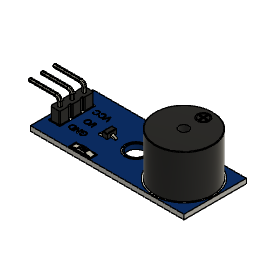
Buzzer (Autodesk Fusion 360 design; units mm, degrees)
Autodesk Fusion 360 part; units mm, degrees
note: some values were not read from the file. Set by a fixed rule: which face or edge a step refers to.
sketch "Sketch1" plane through (0, 0, 0) normal (0, 0, 1) x (1, 0, 0)
  line L0 (16, 6.5) -> (-16, 6.5)
  line L1 (-16, 6.5) -> (-16, -6.5)
  line L2 (-16, -6.5) -> (16, -6.5)
  line L3 (16, -6.5) -> (16, 6.5)
  line L4 (16, 6.5) -> (-16, -6.5) construction
  line L5 (-16, 6.5) -> (16, -6.5) construction
  dimension "d1" = 32
  dimension "d2" = 13
  constraint horizontal L0
  constraint perpendicular L0 L1
  constraint parallel L0 L2
  constraint parallel L1 L3
  constraint coincident L4 origin
  constraint coincident L5 origin
  measures "d1" distance of L1.end L2.end
  measures "d2" distance of L0.end L1.end
extrude "Extrude1" add sketch "Sketch1" along normal blind 1 makes body 1
sketch "Sketch2" plane through (0, 0, 1) normal (0, 0, 1) x (-1, 0, 0)
  line L0 (-16, 6.5) -> (-16, -6.5)
  line L1 (-16, -6.5) -> (16, -6.5)
  line L2 (16, -6.5) -> (16, 6.5)
  line L3 (16, 6.5) -> (-16, 6.5)
  circle A0 centre (-9.5, 0) radius 6
  line L4 (-9.5, 0) -> (-9.5, -6)
  line L5 (-9.5, 0) -> (-15.5, 0)
  circle A1 centre (0.5, 0) radius 1.75
  line L6 (5.5, 1) -> (6.5, 1)
  line L7 (6.5, 1) -> (6.5, -1)
  line L8 (6.5, -1) -> (5.5, -1)
  line L9 (5.5, -1) -> (5.5, 1)
  line L10 (5.5, 1) -> (6.5, -1) construction
  line L11 (6.5, 1) -> (5.5, -1) construction
  line L12 (6.5, 1) -> (7.5, 1)
  line L13 (7.5, 1) -> (7.5, 0.5)
  line L14 (7.5, 0.5) -> (6.5, 0.5)
  line L15 (6.5, 0.5) -> (6.5, 1)
  line L16 (6.5, -1) -> (7.5, -1)
  line L17 (7.5, -1) -> (7.5, -0.5)
  line L18 (7.5, -0.5) -> (6.5, -0.5)
  line L19 (6.5, -0.5) -> (6.5, -1)
  line L20 (5.5, 0.25) -> (4.5, 0.25)
  line L21 (4.5, 0.25) -> (4.5, -0.25)
  line L22 (4.5, -0.25) -> (5.5, -0.25)
  line L23 (5.5, -0.25) -> (5.5, 0.25)
  line L24 (4, 6) -> (8, 6)
  line L25 (8, 6) -> (8, 5)
  line L26 (8, 5) -> (4, 5)
  line L27 (4, 5) -> (4, 6)
  line L28 (6, 0) -> (6, 5.5)
  line L29 (4, 6) -> (5.25, 6)
  line L30 (5.25, 6) -> (5.25, 5)
  line L31 (8, 6) -> (6.75, 6)
  line L32 (6.75, 6) -> (6.75, 5)
  line L33 (14.325, 2.705) -> (13.675, 2.705)
  line L34 (13.675, 2.705) -> (13.675, 2.055)
  line L35 (13.675, 2.055) -> (14.325, 2.055)
  line L36 (14.325, 2.055) -> (14.325, 2.705)
  line L37 (14.325, 2.705) -> (13.675, 2.055) construction
  line L38 (13.675, 2.705) -> (14.325, 2.055) construction
  line L39 (13.675, -0.485) -> (14.325, -0.485)
  line L40 (14.325, -0.485) -> (14.325, 0.165)
  line L41 (14.325, 0.165) -> (13.675, 0.165)
  line L42 (13.675, 0.165) -> (13.675, -0.485)
  line L43 (13.675, -0.485) -> (14.325, 0.165) construction
  line L44 (14.325, -0.485) -> (13.675, 0.165) construction
  line L45 (13.675, -3.025) -> (14.325, -3.025)
  line L46 (14.325, -3.025) -> (14.325, -2.375)
  line L47 (14.325, -2.375) -> (13.675, -2.375)
  line L48 (13.675, -2.375) -> (13.675, -3.025)
  line L49 (13.675, -3.025) -> (14.325, -2.375) construction
  line L50 (14.325, -3.025) -> (13.675, -2.375) construction
  line L51 (15, 1.38) -> (13, 1.38)
  line L52 (13, 1.38) -> (13, 3.38)
  line L53 (13, 3.38) -> (15, 3.38)
  line L54 (15, 3.38) -> (15, 1.38)
  line L55 (15, 1.38) -> (13, 3.38) construction
  line L56 (13, 1.38) -> (15, 3.38) construction
  line L57 (15, -1.16) -> (13, -1.16)
  line L58 (13, -1.16) -> (13, 0.84)
  line L59 (13, 0.84) -> (15, 0.84)
  line L60 (15, 0.84) -> (15, -1.16)
  line L61 (15, -1.16) -> (13, 0.84) construction
  line L62 (13, -1.16) -> (15, 0.84) construction
  line L63 (13.3, 1.38) -> (13.3, 0.84)
  line L64 (14.7, 1.38) -> (14.7, 0.84)
  line L65 (15, -1.7) -> (13, -1.7)
  line L66 (13, -1.7) -> (13, -3.7)
  line L67 (13, -3.7) -> (15, -3.7)
  line L68 (15, -3.7) -> (15, -1.7)
  line L69 (15, -1.7) -> (13, -3.7) construction
  line L70 (13, -1.7) -> (15, -3.7) construction
  line L71 (13.3, -1.16) -> (13.3, -1.7)
  line L72 (14.7, -1.16) -> (14.7, -1.7)
  circle A2 centre (0.5, 0) radius 2
  circle A3 centre (0.5, 0) radius 2.25
  circle A4 centre (-9.5, 0) radius 6.3
  line L73 (4, 6.1) -> (8, 6.1)
  line L74 (8, 4.9) -> (4, 4.9)
  line L75 (8.1, 6) -> (8.1, 5)
  line L76 (3.9, 5) -> (3.9, 6)
  line L77 (3.9, 6) -> (3.9, 6.1)
  line L78 (3.9, 6.1) -> (4, 6.1)
  line L79 (8, 6.1) -> (8.1, 6.1)
  line L80 (8.1, 6.1) -> (8.1, 6)
  line L81 (8, 4.9) -> (8.1, 4.9)
  line L82 (8.1, 4.9) -> (8.1, 5)
  line L83 (3.9, 5) -> (3.9, 4.9)
  line L84 (3.9, 4.9) -> (4, 4.9)
  line L85 (12.8, 1.38) -> (12.8, 3.38)
  line L86 (15.2, 3.38) -> (15.2, 1.38)
  line L87 (12.8, -1.7) -> (12.8, -3.7)
  line L88 (15.2, -3.7) -> (15.2, -1.7)
  line L89 (15.2, 1.38) -> (15.2, -1.7)
  line L90 (12.8, 1.38) -> (12.8, -1.7)
  line L91 (13, 3.58) -> (15, 3.58)
  line L92 (13, -3.9) -> (15, -3.9)
  line L93 (15, -3.9) -> (15.2, -3.9)
  line L94 (15.2, -3.9) -> (15.2, -3.7)
  line L95 (12.8, -3.7) -> (12.8, -3.9)
  line L96 (12.8, -3.9) -> (13, -3.9)
  line L97 (13, 3.58) -> (12.8, 3.58)
  line L98 (12.8, 3.58) -> (12.8, 3.38)
  line L99 (15, 3.58) -> (15.2, 3.58)
  line L100 (15.2, 3.58) -> (15.2, 3.38)
  line L101 (8.25, 6.25) -> (3.75, 6.25)
  line L102 (3.75, 6.25) -> (3.75, 4.75)
  line L103 (3.75, 4.75) -> (8.25, 4.75)
  line L104 (8.25, 4.75) -> (8.25, 6.25)
  line L105 (8.25, 6.25) -> (3.75, 4.75) construction
  line L106 (3.75, 6.25) -> (8.25, 4.75) construction
  line L107 (8.4907, 1.5124) -> (11.9345, 1.5124) construction
  line L108 (11.9345, 1.5124) -> (11.9345, 3.2687) construction
  line L109 (11.9345, 3.2687) -> (8.4907, 3.2687) construction
  line L110 (8.4907, 3.2687) -> (8.4907, 1.5124) construction
  line L111 (8.5, -1.25) -> (12.1, -1.25) construction
  line L112 (12.1, -1.25) -> (12.1, 0.95) construction
  line L113 (12.1, 0.95) -> (8.5, 0.95) construction
  line L114 (8.5, 0.95) -> (8.5, -1.25) construction
  line L115 (8.4, -3.85) -> (12.2, -3.85) construction
  line L116 (12.2, -3.85) -> (12.2, -1.65) construction
  line L117 (12.2, -1.65) -> (8.4, -1.65) construction
  line L118 (8.4, -1.65) -> (8.4, -3.85) construction
  point P0 (6, 0)
  point P1 (5.5, 0)
  point P2 (14, 2.38)
  point P3 (14, -0.16)
  point P4 (14, -2.7)
  point P5 (14, 2.38)
  point P6 (14, -0.16)
  point P7 (14, -2.7)
  point P8 (6, 5.5)
  dimension "d5" = 12
  dimension "d17" = 0.5
  dimension "d18" = 0.5
  dimension "d19" = 3.5
  dimension "d20" = 10
  dimension "d22" = 1
  dimension "d23" = 2
  dimension "d24" = 6
  dimension "d27" = 1
  dimension "d28" = 0.5
  dimension "d29" = 1
  dimension "d30" = 0.5
  dimension "d31" = 1
  dimension "d32" = 0.5
  dimension "d33" = 0.25
  dimension "d36" = 4
  dimension "d37" = 1
  dimension "d38" = 0.5
  dimension "d39" = 1.25
  dimension "d40" = 1.25
  dimension "d81" = 0.65
  dimension "d82" = 0.65
  dimension "d83" = 0.65
  dimension "d84" = 0.65
  dimension "d85" = 2.54
  dimension "d86" = 0.65
  dimension "d87" = 0.65
  dimension "d88" = 2.54
  dimension "d89" = 3.8
  dimension "d90" = 2
  dimension "d91" = 2
  dimension "d92" = 2
  dimension "d93" = 2
  dimension "d94" = 0.3
  dimension "d95" = 0.3
  dimension "d96" = 2
  dimension "d97" = 2
  dimension "d98" = 0.3
  dimension "d99" = 0.3
  dimension "d132" = 4
  dimension "d133" = 4.5
  dimension "d136" = 12.6
  dimension "d137" = -0.1
  dimension "d138" = -0.1
  dimension "d139" = -0.1
  dimension "d140" = -0.1
  dimension "d141" = -0.2
  dimension "d142" = -0.2
  dimension "d143" = 0.2
  dimension "d144" = 0.2
  dimension "d145" = -0.2
  dimension "d146" = 0.2
  dimension "d147" = 4.5
  dimension "d148" = 1.5
  dimension "d197" = 1.15
  dimension "d198" = 1.15
  dimension "d199" = 1.15
  text T0 "GND" font "Arial" height 1.15 align centre middle in box 3.4438 x 1.7563 at (8.4907, 1.5124) x (1, 0) y (0, 1) spacing 1 kerned
  text T1 "I/O" font "Arial" height 1.15 align centre middle in box 3.6 x 2.2 at (8.5, -1.25) x (1, 0) y (0, 1) spacing 1 kerned
  text T2 "VCC" font "Arial" height 1.15 align centre middle in box 3.8 x 2.2 at (8.4, -3.85) x (1, 0) y (0, 1) spacing 1 kerned
  constraint coincident A0.centre L4.start
  constraint coincident A0 L4.end
  constraint vertical L4
  constraint coincident A0 L5.end
  constraint perpendicular L4 L5
  constraint horizontal L6
  constraint perpendicular L6 L7
  constraint parallel L6 L8
  constraint parallel L7 L9
  constraint coincident L10 P0
  constraint coincident L11 P0
  constraint horizontal L12
  constraint vertical L13
  constraint horizontal L14
  constraint vertical L15
  constraint horizontal L16
  constraint vertical L17
  constraint horizontal L18
  constraint vertical L19
  constraint horizontal L20
  constraint vertical L21
  constraint horizontal L22
  constraint vertical L23
  constraint coincident L9 L20.start
  constraint midpoint L9 P1
  constraint horizontal L24
  constraint vertical L25
  constraint horizontal L26
  constraint vertical L27
  constraint coincident P0 L28.start
  constraint perpendicular L26 L28
  constraint perpendicular L27 L29
  constraint coincident L26 L30.end
  constraint perpendicular L26 L30
  constraint perpendicular L25 L31
  constraint coincident L26 L32.end
  constraint perpendicular L26 L32
  constraint horizontal L33
  constraint perpendicular L33 L34
  constraint parallel L33 L35
  constraint parallel L34 L36
  constraint coincident L37 P5
  constraint coincident L38 P5
  constraint horizontal L39
  constraint perpendicular L39 L40
  constraint parallel L39 L41
  constraint parallel L40 L42
  constraint coincident L43 P6
  constraint coincident L44 P6
  constraint horizontal L45
  constraint perpendicular L45 L46
  constraint parallel L45 L47
  constraint parallel L46 L48
  constraint coincident L49 P7
  constraint coincident L50 P7
  constraint horizontal L51
  constraint perpendicular L51 L52
  constraint parallel L51 L53
  constraint parallel L52 L54
  constraint coincident L55 P5
  constraint coincident L56 P5
  constraint coincident P5 P2
  constraint horizontal L57
  constraint perpendicular L57 L58
  constraint parallel L57 L59
  constraint parallel L58 L60
  constraint coincident L61 P6
  constraint coincident L62 P6
  constraint coincident P6 P3
  constraint coincident L51 L63.start
  constraint coincident L59 L63.end
  constraint perpendicular L59 L63
  constraint coincident L51 L64.start
  constraint coincident L59 L64.end
  constraint perpendicular L59 L64
  constraint horizontal L65
  constraint perpendicular L65 L66
  constraint parallel L65 L67
  constraint parallel L66 L68
  constraint coincident L69 P7
  constraint coincident L70 P7
  constraint coincident P7 P4
  constraint coincident L57 L71.start
  constraint coincident L65 L71.end
  constraint perpendicular L65 L71
  constraint coincident L57 L72.start
  constraint coincident L65 L72.end
  constraint perpendicular L65 L72
  constraint concentric A1 A2
  constraint concentric A1 A3
  constraint concentric A0 A4
  constraint parallel L76 L77
  constraint parallel L73 L79
  constraint perpendicular L75 L81
  constraint perpendicular L74 L82
  constraint perpendicular L74 L83
  constraint perpendicular L83 L84
  constraint parallel L92 L93
  constraint parallel L87 L95
  constraint horizontal L97
  constraint horizontal L99
  constraint horizontal L101
  constraint perpendicular L101 L102
  constraint parallel L101 L103
  constraint parallel L102 L104
  constraint coincident L105 P8
  constraint coincident L106 P8
  constraint coincident P8 L28.end
  measures "d5" diameter of A0
  measures "d17" distance of L0 L5.end
  measures "d18" distance of L1 L4.end
  measures "d19" diameter of A1
  measures "d20" distance of A0.centre A1.centre
  measures "d22" distance of L7.end L8.end
  measures "d23" distance of L6.end L7.end
  measures "d24" distance of A1.centre L7
  measures "d27" distance of L6.end L12.end
  measures "d28" distance of L6.end L14.end
  measures "d29" distance of L7.end L16.end
  measures "d30" distance of L7.end L18.end
  measures "d31" distance of L20.start L20.end
  measures "d32" distance of L20.start L22.end
  measures "d33" distance of L20 P1
  measures "d36" distance of L24.start L24.end
  measures "d37" distance of L24.start L26.end
  measures "d38" distance of L3 L24
  measures "d39" distance of L24.start L29.end
  measures "d40" distance of L24.end L31.end
  measures "d81" distance of L34.end L35.end
  measures "d82" distance of L33.end L34.end
  measures "d83" distance of L40.end L41.end
  measures "d84" distance of L39.end L40.end
  measures "d85" distance of P5 P6
  measures "d86" distance of L46.end L47.end
  measures "d87" distance of L45.end L46.end
  measures "d88" distance of P6 P7
  measures "d89" distance of L1 P7
  measures "d90" distance of L52.end L53.end
  measures "d91" distance of L51.end L52.end
  measures "d92" distance of L58.end L59.end
  measures "d93" distance of L57.end L58.end
  measures "d94" distance of L51.end L63
  measures "d95" distance of L51.start L64
  measures "d96" distance of L66.end L67.end
  measures "d97" distance of L65.end L66.end
  measures "d98" distance of L57.end L71
  measures "d99" distance of L57.start L72
  measures "d132" diameter of A2
  measures "d133" diameter of A3
  measures "d136" diameter of A4
  measures "d147" distance of L102.end L103.end
  measures "d148" distance of L101.end L102.end
extrude "Extrude2" add sketch "Sketch2" along normal blind 9 contours A0 L4 L5 | A0 L4 L5 bodies 1
sketch "Sketch3" plane through (0, 0, 10) normal (0, 0, 1) x (-1, 0, 0)
  circle A0 centre (-9.5, 0) radius 6
  circle A1 centre (-9.5, 0) radius 1
  dimension "d11" = 2
  constraint concentric A0 A1
  measures "d11" diameter of A1
extrude "Extrude3" cut sketch "Sketch3" against normal blind 5 contours A1 bodies 1
extrude "Extrude4" cut sketch "Sketch2" against normal through all contours A1 bodies 1
extrude "Extrude5" add sketch "Sketch2" along normal blind 1 contours L6 L7 L8 L9 L15 L19 L23 bodies 1
extrude "Extrude6" add sketch "Sketch2" along normal blind 0.5 separate body contours L9 L20 L21 L22 L23 | L7 L12 L13 L14 L15 | L7 L16 L17 L18 L19 makes body 2 at (-4.8333, 0.25, 1.1667) makes body 3 at (-6.8333, -1, 1.1667) makes body 4 at (-6.8333, 1, 1.1667)
extrude "Extrude7" add sketch "Sketch2" along normal blind 0.5 contours L24 L26 L30 L32 bodies 3 2 4 1
extrude "Extrude8" add sketch "Sketch2" along normal blind 0.25 contours L24 L26 L27 L29 L30 | L24 L25 L26 L31 L32 bodies 1 2 4 3
extrude "Extrude10" add sketch "Sketch2" along normal blind 2.5 contours L33 L34 L35 L36 | L39 L40 L41 L42 | L45 L46 L47 L48 | L51 L52 L53 L54 | L51 L59 L63 L64 | L57 L58 L59 L60 | L57 L65 L71 L72 | L65 L66 L67 L68 bodies 1 3 4 2
extrude "Extrude11" add sketch "Sketch2" along normal blind 4.5 contours L33 L34 L35 L36 | L39 L40 L41 L42 | L45 L46 L47 L48 bodies 3 2 4 1
sketch "Sketch6" plane through (-14.325, 0, 0) normal (-1, 0, 0) x (0, -1, 0)
  line L0 (-3.025, 3.5) -> (-2.375, 3.5)
  line L1 (-2.375, 3.5) -> (-2.375, 5.5)
  line L2 (-2.375, 5.5) -> (-3.025, 5.5)
  line L3 (-3.025, 5.5) -> (-3.025, 3.5)
  line L4 (-3.025, 5.5) -> (-2.375, 5.5)
  line L5 (-2.375, 5.5) -> (-2.375, 4.85)
  line L6 (-2.375, 4.85) -> (-3.025, 4.85)
  line L7 (-3.025, 4.85) -> (-3.025, 5.5)
  dimension "d104" = 0.65
  dimension "d105" = 0.65
  constraint horizontal L4
  constraint vertical L5
  constraint horizontal L6
  constraint vertical L7
  constraint coincident L2.end L3.start
  measures "d104" distance of L2.end L1.end
  measures "d105" distance of L2.end L6.end
sketch "Sketch7" plane through (-14.325, 0, 0) normal (-1, 0, 0) x (0, -1, 0)
  line L0 (-0.485, 3.5) -> (0.165, 3.5)
  line L1 (0.165, 3.5) -> (0.165, 5.5)
  line L2 (0.165, 5.5) -> (-0.485, 5.5)
  line L3 (-0.485, 5.5) -> (-0.485, 3.5)
  line L4 (-0.485, 5.5) -> (0.165, 5.5)
  line L5 (0.165, 5.5) -> (0.165, 4.85)
  line L6 (0.165, 4.85) -> (-0.485, 4.85)
  line L7 (-0.485, 4.85) -> (-0.485, 5.5)
  dimension "d108" = 0.65
  dimension "d109" = 0.65
  constraint horizontal L4
  constraint vertical L5
  constraint horizontal L6
  constraint vertical L7
  constraint coincident L2.end L3.start
  measures "d108" distance of L2.end L1.end
  measures "d109" distance of L2.end L6.end
sketch "Sketch8" plane through (-14.325, 0, 0) normal (-1, 0, 0) x (0, -1, 0)
  line L0 (2.055, 3.5) -> (2.705, 3.5)
  line L1 (2.705, 3.5) -> (2.705, 5.5)
  line L2 (2.705, 5.5) -> (2.055, 5.5)
  line L3 (2.055, 5.5) -> (2.055, 3.5)
  line L4 (2.055, 5.5) -> (2.705, 5.5)
  line L5 (2.705, 5.5) -> (2.705, 4.85)
  line L6 (2.705, 4.85) -> (2.055, 4.85)
  line L7 (2.055, 4.85) -> (2.055, 5.5)
  dimension "d110" = 0.65
  dimension "d111" = 0.65
  constraint horizontal L4
  constraint vertical L5
  constraint horizontal L6
  constraint vertical L7
  constraint coincident L2.end L3.start
  measures "d110" distance of L2.end L1.end
  measures "d111" distance of L2.end L6.end
extrude "Extrude13" add sketch "Sketch6" sketch "Sketch8" sketch "Sketch7" along normal blind 6 contours L1 L2 L3 L4 L5 L6 L7 of sketch 2 contours L1 L2 L3 L4 L5 L6 L7 of sketch 3 contours L1 L2 L3 L4 L5 L6 L7 bodies 4 2 1 3
fillet "Fillet1" radius 0.1 1 edges at (15.094, 2.1697, 10) on bodies 1
fillet "Fillet2" radius 10 2 edges at (-8, -5.5, 1.25) (-4, -5.5, 1.25) on bodies 1
fillet "Fillet3" radius 0.1 4 edges at (-6.75, -5.5, 1.5) (-6, -5, 1.5) (-5.25, -5.5, 1.5) (-6, -6, 1.5) on bodies 1
fillet "Fillet4" radius 0.1 4 edges at (-6.5, 0, 2) (-5.5, 0, 2) (-6, -1, 2) (-6, 1, 2) on bodies 1
fillet "Fillet5" radius 2 3 edges at (-7.5, 0.75, 1.5) (-7.5, -0.75, 1.5) (-4.5, 0, 1.5) on bodies 2 3 4
fillet "Fillet6" radius 0.2 12 edges at (-15, 3.7, 2.25) (-13, 3.7, 2.25) (-13, 1.7, 2.25) (-13, -1.38, 2.25) (-13, -0.84, 2.25) (-13, -3.38, 2.25) (-15, -3.38, 2.25) (-15, -1.38, 2.25) (-15, -0.84, 2.25) (-15, 1.16, 2.25) (-15, 1.7, 2.25) (-13, 1.16, 2.25) on bodies 1
fillet "Fillet7" radius 1 3 edges at (-13.675, 2.7, 5.5) (-13.675, 0.16, 5.5) (-13.675, -2.38, 5.5) on bodies 1
fillet "Fillet8" radius 0.5 3 edges at (-14.325, 2.7, 4.85) (-14.325, 0.16, 4.85) (-14.325, -2.38, 4.85) on bodies 1
fillet "Fillet9" radius 0.2 48 edges at (-13.675, 0.485, 4) (-13.9679, 0.485, 5.2071) (-17.5, 0.485, 5.5) (-14.325, 2.375, 3.925) (-14.4714, 2.375, 4.7036) (-17.575, 2.375, 4.85) (-13.675, -0.165, 4) (-13.9679, -0.165, 5.2071) (-17.5, -0.165, 5.5) (-14.325, -2.055, 3.925) (-14.4714, -2.055, 4.7036) (-17.575, -2.055, 4.85) (-20.325, -2.38, 5.5) (-14.325, -0.165, 3.925) (-14.4714, -0.165, 4.7036) (-17.575, -0.165, 4.85) (-13.675, -2.055, 4) (-13.9679, -2.055, 5.2071) (-17.5, -2.055, 5.5) (-20.325, 3.025, 5.175) (-20.325, 2.375, 5.175) (-20.325, -2.705, 5.175) (-20.325, 0.485, 5.175) (-13.675, 3.025, 4) (-13.9679, 3.025, 5.2071) (-17.5, 3.025, 5.5) (-17.5, -2.705, 5.5) (-13.9679, -2.705, 5.2071) (-13.675, -2.705, 4) (-17.575, 3.025, 4.85) (-14.4714, 3.025, 4.7036) (-14.325, 3.025, 3.925) (-20.325, 0.16, 5.5) (-20.325, -2.38, 4.85) (-20.325, 2.7, 4.85) (-14.325, 0.485, 3.925) (-14.4714, 0.485, 4.7036) (-17.575, 0.485, 4.85) (-20.325, -2.055, 5.175) (-20.325, 2.7, 5.5) (-20.325, 0.16, 4.85) (-13.675, 2.375, 4) (-13.9679, 2.375, 5.2071) (-17.5, 2.375, 5.5) (-14.325, -2.705, 3.925) (-14.4714, -2.705, 4.7036) (-17.575, -2.705, 4.85) (-20.325, -0.165, 5.175) on bodies 1
sketch "Sketch9" plane through (0, 1, 0) normal (0, 1, 0) x (-1, 0, 0)
  line L0 (6.5, 1) -> (6.5, 1.9)
  line L1 (6.5, 1.9) -> (5.5, 1.9)
  line L2 (5.5, 1.9) -> (5.5, 1)
  line L3 (5.5, 1) -> (6.5, 1)
extrude "Extrude14" add sketch "Sketch2" along normal blind 0.01 contours A3 | A4 | L85 L86 L87 L88 L89 L90 L91 L92 L93 L94 L95 L96 L97 L98 L99 L100 | L101 L102 L103 L104 bodies 1
sketch "Sketch10" plane through (0, 0, 0) normal (0, 0, -1) x (1, 0, 0)
  circle A0 centre (-0.5, 0) radius 1.75
  line L0 (16, -6.5) -> (16, 6.5)
  line L1 (16, 6.5) -> (-16, 6.5)
  line L2 (-16, 6.5) -> (-16, -6.5)
  line L3 (-16, -6.5) -> (16, -6.5)
  circle A1 centre (-14, -2.7) radius 1
  circle A2 centre (-14, -0.16) radius 1
  circle A3 centre (-14, -2.7) radius 1.15
  circle A4 centre (-14, -0.16) radius 1.15
  circle A5 centre (-14, 2.38) radius 1.15
  circle A6 centre (-14, 2.38) radius 1
  line L4 (-14.325, -2.375) -> (-13.675, -2.375)
  line L5 (-13.675, -2.375) -> (-13.675, -3.025)
  line L6 (-13.675, -3.025) -> (-14.325, -3.025)
  line L7 (-14.325, -3.025) -> (-14.325, -2.375)
  line L8 (-14.325, -2.375) -> (-13.675, -3.025) construction
  line L9 (-13.675, -2.375) -> (-14.325, -3.025) construction
  line L10 (-14.325, 0.165) -> (-13.675, 0.165)
  line L11 (-13.675, 0.165) -> (-13.675, -0.485)
  line L12 (-13.675, -0.485) -> (-14.325, -0.485)
  line L13 (-14.325, -0.485) -> (-14.325, 0.165)
  line L14 (-14.325, 0.165) -> (-13.675, -0.485) construction
  line L15 (-13.675, 0.165) -> (-14.325, -0.485) construction
  line L16 (-14.325, 2.705) -> (-13.675, 2.705)
  line L17 (-13.675, 2.705) -> (-13.675, 2.055)
  line L18 (-13.675, 2.055) -> (-14.325, 2.055)
  line L19 (-14.325, 2.055) -> (-14.325, 2.705)
  line L20 (-14.325, 2.705) -> (-13.675, 2.055) construction
  line L21 (-13.675, 2.705) -> (-14.325, 2.055) construction
  point P0 (-14, -0.16)
  point P1 (-14, -2.7)
  point P2 (-14, 2.38)
  point P3 (-14, -2.7)
  point P4 (-14, -0.16)
  point P5 (-14, 2.38)
  dimension "d149" = 2
  dimension "d150" = 2
  dimension "d171" = 2.3
  dimension "d172" = 2.3
  dimension "d182" = 2.3
  dimension "d183" = 2
  dimension "d202" = 0.65
  dimension "d203" = 0.65
  dimension "d204" = 0.65
  dimension "d205" = 0.65
  dimension "d206" = 0.65
  dimension "d207" = 0.65
  constraint coincident P3 P1
  constraint coincident P4 P0
  constraint coincident P5 P2
  constraint concentric A5 A6
  constraint horizontal L4
  constraint perpendicular L4 L5
  constraint parallel L4 L6
  constraint parallel L5 L7
  constraint coincident L8 P3
  constraint coincident L9 P3
  constraint horizontal L10
  constraint perpendicular L10 L11
  constraint parallel L10 L12
  constraint parallel L11 L13
  constraint coincident L14 P4
  constraint coincident L15 P4
  constraint horizontal L16
  constraint perpendicular L16 L17
  constraint parallel L16 L18
  constraint parallel L17 L19
  constraint coincident L20 P5
  constraint coincident L21 P5
  measures "d149" diameter of A1
  measures "d150" diameter of A2
  measures "d171" diameter of A3
  measures "d172" diameter of A4
  measures "d182" diameter of A5
  measures "d183" diameter of A6
  measures "d202" distance of L5.end L6.end
  measures "d203" distance of L4.end L5.end
  measures "d204" distance of L11.end L12.end
  measures "d205" distance of L10.end L11.end
  measures "d206" distance of L17.end L18.end
  measures "d207" distance of L16.end L17.end
extrude "Extrude15" add sketch "Sketch10" along normal blind 1.5 contours L4 L5 L6 L7 | L10 L11 L12 L13 | L16 L17 L18 L19 bodies 1
loft "Loft1" add profiles "Sketch10" section 1 face at (-14.1083, 2.5917, -1.5) section 2 contours A1 | L4 L5 L6 L7 on bodies 1 bodies 1
loft "Loft2" add profiles "Sketch10" section 1 contours A2 | L10 L11 L12 L13 section 2 face at (-13.8917, 0.2683, -1.5) on bodies 1 bodies 1
loft "Loft6" add profiles "Sketch10" section 1 face at (-14.1083, -2.4883, -1.5) section 2 contours A6 on bodies 1 bodies 1
sketch "Sketch11" plane through (0, 0, 0) normal (0, 0, -1) x (1, 0, 0)
  circle A0 centre (-0.5, 0) radius 1.75
  line L0 (16, -6.5) -> (16, 6.5)
  line L1 (16, 6.5) -> (-16, 6.5)
  line L2 (-16, 6.5) -> (-16, -6.5)
  line L3 (-16, -6.5) -> (16, -6.5)
  circle A1 centre (9.5, -3.5) radius 1
  circle A2 centre (9.5, -3.5) radius 0.35
  line L4 (10.5, 2.5) -> (8.5, 2.5)
  line L5 (8.5, 2.5) -> (8.5, 4.5)
  line L6 (8.5, 4.5) -> (10.5, 4.5)
  line L7 (10.5, 4.5) -> (10.5, 2.5)
  line L8 (10.5, 2.5) -> (8.5, 4.5) construction
  line L9 (8.5, 2.5) -> (10.5, 4.5) construction
  line L10 (9.85, 3.15) -> (9.15, 3.15)
  line L11 (9.15, 3.15) -> (9.15, 3.85)
  line L12 (9.15, 3.85) -> (9.85, 3.85)
  line L13 (9.85, 3.85) -> (9.85, 3.15)
  line L14 (9.85, 3.15) -> (9.15, 3.85) construction
  line L15 (9.15, 3.15) -> (9.85, 3.85) construction
  line L16 (10.75, 2.25) -> (8.25, 2.25)
  line L17 (8.25, 2.25) -> (8.25, 4.75)
  line L18 (8.25, 4.75) -> (10.75, 4.75)
  line L19 (10.75, 4.75) -> (10.75, 2.25)
  line L20 (10.75, 2.25) -> (8.25, 4.75) construction
  line L21 (8.25, 2.25) -> (10.75, 4.75) construction
  circle A3 centre (9.5, -3.5) radius 1.2
  spline S0 degree 3 poles (-13.2929, 0.5471) (-13.11, 0.3642) (-13.0025, 0.1082) (-13, -0.1504) (-12.9975, -0.4154) (-13.1055, -0.6797) (-13.2929, -0.8671) knots -1 -1 -1 -1 -0.506107 -0.506107 -0.506107 0 0 0 0
  spline S1 degree 3 poles (-13.2929, -0.8671) (-13.4758, -1.05) (-13.7318, -1.1575) (-13.9904, -1.16) (-14.2554, -1.1625) (-14.5197, -1.0545) (-14.7071, -0.8671) knots -1 -1 -1 -1 -0.506107 -0.506107 -0.506107 0 0 0 0
  spline S2 degree 3 poles (-14.7071, -0.8671) (-14.89, -0.6842) (-14.9975, -0.4282) (-15, -0.1696) (-15.0025, 0.0954) (-14.8945, 0.3597) (-14.7071, 0.5471) knots -1 -1 -1 -1 -0.506107 -0.506107 -0.506107 0 0 0 0
  spline S3 degree 3 poles (-14.7071, 0.5471) (-14.5242, 0.73) (-14.2682, 0.8375) (-14.0096, 0.84) (-13.7446, 0.8425) (-13.4803, 0.7345) (-13.2929, 0.5471) knots -1 -1 -1 -1 -0.506107 -0.506107 -0.506107 0 0 0 0
  spline S4 degree 3 poles (-14.7071, -3.4071) (-14.8945, -3.2197) (-15.0025, -2.9554) (-15, -2.6904) (-14.9975, -2.4318) (-14.89, -2.1758) (-14.7071, -1.9929) knots 0 0 0 0 0.506107 0.506107 0.506107 1 1 1 1
  spline S5 degree 3 poles (-14.7071, -1.9929) (-14.5197, -1.8055) (-14.2554, -1.6975) (-13.9904, -1.7) (-13.7318, -1.7025) (-13.4758, -1.81) (-13.2929, -1.9929) knots 0 0 0 0 0.506107 0.506107 0.506107 1 1 1 1
  spline S6 degree 3 poles (-13.2929, -1.9929) (-13.1055, -2.1803) (-12.9975, -2.4446) (-13, -2.7096) (-13.0025, -2.9682) (-13.11, -3.2242) (-13.2929, -3.4071) knots 0 0 0 0 0.506107 0.506107 0.506107 1 1 1 1
  spline S7 degree 3 poles (-13.2929, -3.4071) (-13.4803, -3.5945) (-13.7446, -3.7025) (-14.0096, -3.7) (-14.2682, -3.6975) (-14.5242, -3.59) (-14.7071, -3.4071) knots 0 0 0 0 0.506107 0.506107 0.506107 1 1 1 1
  spline S8 degree 3 poles (-14.7071, 1.6729) (-14.8945, 1.8603) (-15.0025, 2.1246) (-15, 2.3896) (-14.9975, 2.6482) (-14.89, 2.9042) (-14.7071, 3.0871) knots 0 0 0 0 0.506107 0.506107 0.506107 1 1 1 1
  spline S9 degree 3 poles (-14.7071, 3.0871) (-14.5197, 3.2745) (-14.2554, 3.3825) (-13.9904, 3.38) (-13.7318, 3.3775) (-13.4758, 3.27) (-13.2929, 3.0871) knots 0 0 0 0 0.506107 0.506107 0.506107 1 1 1 1
  spline S10 degree 3 poles (-13.2929, 3.0871) (-13.1055, 2.8997) (-12.9975, 2.6354) (-13, 2.3704) (-13.0025, 2.1118) (-13.11, 1.8558) (-13.2929, 1.6729) knots 0 0 0 0 0.506107 0.506107 0.506107 1 1 1 1
  spline S11 degree 3 poles (-13.2929, 1.6729) (-13.4803, 1.4855) (-13.7446, 1.3775) (-14.0096, 1.38) (-14.2682, 1.3825) (-14.5242, 1.49) (-14.7071, 1.6729) knots 0 0 0 0 0.506107 0.506107 0.506107 1 1 1 1
  point P0 (9.5, 3.5)
  point P1 (9.5, 3.5)
  point P2 (9.5, 3.5)
  dimension "d159" = 2
  dimension "d160" = 3
  dimension "d161" = 6.5
  dimension "d162" = 0.7
  dimension "d163" = 2
  dimension "d164" = 2
  dimension "d165" = 6.5
  dimension "d166" = 3
  dimension "d167" = 0.7
  dimension "d168" = 0.7
  dimension "d173" = 2.5
  dimension "d174" = 2.5
  dimension "d175" = 2.4
  constraint concentric A1 A2
  constraint horizontal L4
  constraint perpendicular L4 L5
  constraint parallel L4 L6
  constraint parallel L5 L7
  constraint coincident L8 P2
  constraint coincident L9 P2
  constraint horizontal L10
  constraint perpendicular L10 L11
  constraint parallel L10 L12
  constraint parallel L11 L13
  constraint coincident L14 P2
  constraint coincident L15 P2
  constraint coincident P2 P1
  constraint horizontal L16
  constraint perpendicular L16 L17
  constraint parallel L16 L18
  constraint parallel L17 L19
  constraint coincident L20 P2
  constraint coincident L21 P2
  constraint concentric A1 A3
  measures "d159" diameter of A1
  measures "d160" distance of L3 A1.centre
  measures "d161" distance of L0 A1.centre
  measures "d162" diameter of A2
  measures "d163" distance of L5.end L6.end
  measures "d164" distance of L4.end L5.end
  measures "d165" distance of L0 P2
  measures "d166" distance of L1 P2
  measures "d167" distance of L11.end L12.end
  measures "d168" distance of L10.end L11.end
  measures "d173" distance of L17.end L18.end
  measures "d174" distance of L16.end L17.end
  measures "d175" diameter of A3
extrude "Extrude17" add sketch "Sketch11" along normal blind 1 contours A2 | L10 L11 L12 L13 bodies 1
loft "Loft3" add profiles "Sketch11" section 1 contours L4 L5 L6 L7 section 2 face at (9.6167, -3.3833, -1) on bodies 1 bodies 1
loft "Loft4" add profiles "Sketch11" section 1 contours A1 section 2 face at (9.3453, 3.5353, -1) on bodies 1 bodies 1
extrude "Extrude18" cut sketch "Sketch11" sketch "Sketch10" against normal blind 0.2 contours L16 L17 L18 L19 | A3 of sketch 2 contours A3 | A4 | A5 bodies 1
sketch "Sketch12" plane through (0, 0, 10) normal (0, 0, 1) x (-1, 0, 0)
  circle A0 centre (-9.5, 0) radius 1
  circle A1 centre (-9.5, 0) radius 5.9
  circle A2 centre (-9.5575, -3.9997) radius 1
  circle A3 centre (-9.5575, -3.9997) radius 1.25
  line L0 (-9.6825, -3.1997) -> (-9.4325, -3.1997)
  line L1 (-9.4325, -3.1997) -> (-9.4325, -4.7997)
  line L2 (-9.4325, -4.7997) -> (-9.6825, -4.7997)
  line L3 (-9.6825, -4.7997) -> (-9.6825, -3.1997)
  line L4 (-9.6825, -3.1997) -> (-9.4325, -4.7997) construction
  line L5 (-9.4325, -3.1997) -> (-9.6825, -4.7997) construction
  line L6 (-10.3575, -4.1247) -> (-8.7575, -4.1247)
  line L7 (-8.7575, -4.1247) -> (-8.7575, -3.8747)
  line L8 (-8.7575, -3.8747) -> (-10.3575, -3.8747)
  line L9 (-10.3575, -3.8747) -> (-10.3575, -4.1247)
  line L10 (-10.3575, -4.1247) -> (-8.7575, -3.8747) construction
  line L11 (-8.7575, -4.1247) -> (-10.3575, -3.8747) construction
  point P0 (-9.5575, -5.8997)
  point P1 (-9.5575, -3.9997)
  point P2 (-9.5575, -3.9997)
  dimension "d187" = 2
  dimension "d188" = 1.9
  dimension "d190" = 2.5
  dimension "d191" = 0.25
  dimension "d192" = 1.6
  dimension "d193" = 1.6
  dimension "d194" = 0.25
  constraint coincident A1 P0
  constraint concentric A2 A3
  constraint horizontal L0
  constraint perpendicular L0 L1
  constraint parallel L0 L2
  constraint parallel L1 L3
  constraint coincident L4 P2
  constraint coincident L5 P2
  constraint coincident P2 P1
  constraint horizontal L6
  constraint perpendicular L6 L7
  constraint parallel L6 L8
  constraint parallel L7 L9
  constraint coincident L10 P2
  constraint coincident L11 P2
  measures "d187" diameter of A2
  measures "d188" distance of P1 P0
  measures "d190" diameter of A3
  measures "d191" distance of L1.end L2.end
  measures "d192" distance of L0.end L1.end
  measures "d193" distance of L7.end L8.end
  measures "d194" distance of L6.end L7.end
extrude "Extrude21" cut sketch "Sketch12" against normal blind 0.05 contours A3 | L0 L1 L3 L8 | L1 L3 L6 L8 | L3 L6 L8 L9 | L1 L6 L7 L8 | L1 L2 L3 L6 bodies 1
extrude "Extrude22" add sketch "Sketch2" along normal blind 0.005 text T0 T1 T2 bodies 1
sketch "Sketch13" plane through (0, 0, 1.5) normal (0, 0, 1) x (-1, 0, 0)
  line L0 (5.35, 5.9) -> (5.35, 5.1)
  line L1 (5.35, 5.1) -> (6.65, 5.1)
  line L2 (6.65, 5.1) -> (6.65, 5.9)
  line L3 (6.65, 5.9) -> (5.35, 5.9)
  line L4 (5.3955, 5.2052) -> (6.5955, 5.2052) construction
  line L5 (6.5955, 5.2052) -> (6.5955, 5.8052) construction
  line L6 (6.5955, 5.8052) -> (5.3955, 5.8052) construction
  line L7 (5.3955, 5.8052) -> (5.3955, 5.2052) construction
  dimension "d208" = 0.4
  text T0 "102" font "Arial" height 0.4 align centre middle in box 1.2 x 0.6 at (5.3955, 5.2052) x (1, 0) y (0, 1) spacing 1 kerned
extrude "Extrude23" add sketch "Sketch13" along normal blind 0.005 text T0 bodies 1
equation "d95 = d94"
equation "d98 = d95"
equation "d99 = d98"
equation "d165 = d161"
equation "d166 = d160"
